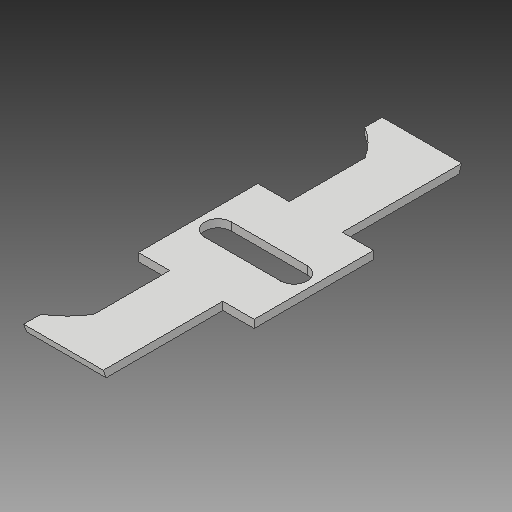
# Autodesk Inventor part: Deslizador
Saved by Autodesk Inventor 2017 (Build 210142000, 142)
## iProperties
Created: 2017-01-19
Part Number: Deslizador
Material: Generic
Document SubType Name: Modeling
Designer: A. Matías Quezada
Density: 1 g/cm^3
Appearance: Default
Author: A. Matías Quezada
Autodesk Inventor part; units mm, degrees
ref_plane "YZ Plane" through (0, 0, 0) normal (1, 0, 0) x (0, 1, 0)
ref_plane "XZ Plane" through (0, 0, 0) normal (0, 1, 0) x (-1, 0, 0)
ref_plane "XY Plane" through (0, 0, 0) normal (0, 0, 1) x (1, 0, 0)
sketch "Sketch1" plane through (0, 0, 0) normal (0, 0, 1) x (1, 0, 0)
  line L0 (0, 0) -> (0, 30)
  line L1 (0, 30) -> (-6.5, 30)
  line L2 (0, 0) -> (-45, 0)
  line L3 (-45, 0) -> (-45, -11.8)
  line L4 (-45, -11.8) -> (-67.5, -11.8)
  line L5 (-67.5, -11.8) -> (-67.5, 31.8)
  line L6 (-67.5, 31.8) -> (-45, 31.8)
  line L7 (-45, 31.8) -> (-45, 20)
  line L8 (-45, 20) -> (-16.5, 20)
  arc A0 (-16.5, 20) -> (-6.5, 30) centre (-32.1155, 45.6155) ccw
  line L9 (-135, 0) -> (-135, 30)
  line L10 (-135, 30) -> (-128.5, 30)
  line L11 (-135, 0) -> (-90, 0)
  line L12 (-90, 0) -> (-90, -11.8)
  line L13 (-90, -11.8) -> (-67.5, -11.8)
  line L14 (-67.5, 31.8) -> (-90, 31.8)
  line L15 (-90, 31.8) -> (-90, 20)
  line L16 (-90, 20) -> (-118.5, 20)
  arc A1 (-128.5, 30) -> (-118.5, 20) centre (-102.8845, 45.6155) ccw
  dimension "d16" = 10
  dimension "d17" = 30
  dimension "d18" = 6.5
  dimension "d19" = 10
  dimension "d20" = 20
  dimension "d23" = 45
  dimension "d24" = 135
  dimension "d25" = 43.6
  constraints: 34 end point, 9 symmetric about line, 7 perpendicular, 4 point on circle, 2 centre point, 2 equal length, 1 horizontal, 1 vertical, 1 other
  measures "d16" horizontal distance of L1.end L8.end
  measures "d17" radius of A0
  measures "d18" distance of L0.end L1.end
  measures "d19" distance between parallel lines of L1 L8
  measures "d20" distance between parallel lines of L11 L16
  measures "d23" distance between parallel lines of L7 L15
  measures "d24" distance between parallel lines of L0 L9
  measures "d25" distance between parallel lines of L13 L14
extrude "Body" add sketch "Sketch1" along normal blind 3
sketch "Sketch2" plane through (0, 0, 3) normal (0, 0, 1) x (1, 0, 0)
  line L0 (-72.5, -4.3) -> (-72.5, 24.3)
  arc A0 (-62.5, 24.3) -> (-72.5, 24.3) centre (-67.5, 24.3) ccw
  line L1 (-62.5, 24.3) -> (-62.5, -4.3)
  arc A1 (-72.5, -4.3) -> (-62.5, -4.3) centre (-67.5, -4.3) ccw
  line L2 (-16.5, 20) -> (-45, 20) projected
  line L3 (0, 0) -> (0, 30) projected
  line L4 (-45, -11.8) -> (-45, 0) projected
  line L5 (-45, 20) -> (-45, 0)
  line L6 (-131.212, 10) -> (6.3115, 10)
  point P0 (-62.5, 10)
  point P1 (-45, 10)
  dimension "d28" = 28.6
  dimension "d30" = 62.5
  dimension "d31" = 10
  constraints: 8 end point, 4 point on circle, 4 tangent, 2 centre point, 2 midpoint, 2 point on line, 2 vertical, 1 collinear, 1 horizontal
  measures "d28" distance of A0.centre A1.centre
  measures "d30" distance between parallel lines of L3 L1
  measures "d31" distance between parallel lines of L1 L0
extrude "Extrusion2" cut sketch "Sketch2" against normal through all
draft "FaceDraft1" angle -20 pull direction (0, 0, 1) faces at (0, 10, 1) fixed edges at (0, 15, 3)
draft "FaceDraft2" angle -20 pull direction (0, 0, 1) faces at (-135, 20, 1) fixed edges at (-135, 15, 3)
equation "\"d16\" = deslizador_interruptor_largo"
equation "\"d17\" = deslizador_interruptor_angulo"
equation "\"d18\" = deslizador_interruptor_separacion"
equation "\"d19\" = deslizador_interruptor_ancho"
equation "\"d20\" = deslizador_ancho"
equation "\"d23\" = deslizador_apoyo_largo"
equation "\"d24\" = deslizador_largo"
equation "\"d25\" = deslizador_ancho + 2 * deslizador_apoyo_ancho"
equation "\"d26\" = deslizador_grosor"
equation "\"d28\" = deslizador_eje_movimiento"
equation "\"d30\" = deslizador_eje_separacion"
equation "\"d31\" = deslizador_eje_ancho"
equation "\"d34\" = tirador_deslizador_agarre"
equation "\"d35\" = tirador_deslizador_agarre"
equation "\"deslizador_interruptor_largo\" = 10"
equation "\"deslizador_interruptor_angulo\" = 30"
equation "\"deslizador_interruptor_separacion\" = 6.5"
equation "\"deslizador_interruptor_ancho\" = 10"
equation "\"deslizador_ancho\" = 20"
equation "\"deslizador_apoyo_largo\" = 45"
equation "\"deslizador_largo\" = 135"
equation "\"deslizador_apoyo_ancho\" = 11.8"
equation "\"deslizador_grosor\" = 3"
equation "\"deslizador_eje_movimiento\" = 28.6"
equation "\"deslizador_eje_separacion\" = 62.5"
equation "\"deslizador_eje_ancho\" = 10"
equation "\"tirador_deslizador_agarre\" = -20deg"
body "Solid1"
